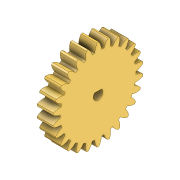
# Autodesk Inventor part: 바퀴 스퍼기어
Saved by Autodesk Inventor 2020 (Build 240168000, 168)
## iProperties
Created: 2020-05-04
Part Number: 바퀴 스퍼기어
Material: 일반
Document SubType Name: Modeling
Designer: sbahn
Density: 1 g/cm^3
Appearance: PTFE
Author: sbahn
## iProperties of the stored document _3D 인쇄.ipt
Created: 2020-06-04
Part Number: _3D 인쇄
Material: 일반
Document SubType Name: Modeling
Designer: Miji
Density: 1 g/cm^3
Appearance: 기본값
Author: Miji
Autodesk Inventor part; units mm, degrees
ref_plane "YZ Plane" through (0, 0, 0) normal (1, 0, 0) x (0, 1, 0)
ref_plane "XZ Plane" through (0, 0, 0) normal (0, 1, 0) x (-1, 0, 0)
ref_plane "XY Plane" through (0, 0, 0) normal (0, 0, 1) x (1, 0, 0)
sketch "스케치1" plane through (0, 0, 0) normal (1, 0, 0) x (0, 1, 0)
  circle A0 centre (0, 0) radius 13 construction
  circle A1 centre (0, 0) radius 14 construction
  circle A2 centre (0, 0) radius 11.75
  line L0 (11.75, 0) -> (14, 0) construction
  line L1 (13.9971, 0.285) -> (11.7465, 0.285) construction
  line L2 (13.978, 0.785) -> (11.7237, 0.785) construction
  line L3 (13.9617, 1.035) -> (11.7043, 1.035) construction
  arc A3 (13.9971, -0.285) -> (13.9971, 0.285) centre (0, 0) ccw
  arc A4 (11.7043, -1.035) -> (11.7043, 1.035) centre (0, 0) ccw
  arc A5 (13.9971, 0.285) -> (11.7043, 1.035) centre (11.4488, -3.6255) ccw
  arc A6 (11.7043, -1.035) -> (13.9971, -0.285) centre (11.4488, 3.6255) ccw
  point P0 (11.7043, -1.035)
  dimension "d0" = 26
  dimension "d2" = 2.25
  dimension "d3" = 0.5
  dimension "d4" = 0.25
  dimension "d5" = 0.785
  dimension "d17" = 1
  constraints: 18 point on circle, 8 end point, 7 centre point, 4 horizontal, 3 symmetric about line, 1 coincident, 1 other
  measures "d0" diameter of A0
  measures "d2" radial gap between concentric circles of A1 A2
  measures "d3" distance between parallel lines of L2 L1
  measures "d4" distance between parallel lines of L3 L2
  measures "d5" distance between parallel lines of L0 L2
  measures "d17" radial gap between concentric circles of A0 A1
extrude "돌출1" add sketch "스케치1" along normal blind 5 contours A2
extrude "돌출2" add sketch "스케치1" along normal blind 5
pattern_circular "원형 패턴1" count 26 over 360 about axis through (0, 0, 0) along (1, 0, 0) of "돌출2"
sketch "스케치2" plane through (5, 0, 0) normal (1, 0, 0) x (0, 0, -1)
  circle A0 centre (0, 0) radius 1.5
  line L0 (0, -1.5) -> (0, 1)
  line L1 (-1.118, 1) -> (1.118, 1)
  dimension "d13" = 3
  dimension "d14" = 2.5
  constraints: 4 end point, 3 point on circle, 1 centre point, 1 coincident, 1 horizontal, 1 vertical
  measures "d13" diameter of A0
  measures "d14" distance of L0.start L0.end
extrude "돌출3" cut sketch "스케치2" against normal blind 5 contours A0 L0 L1 | A0 L1 L0
